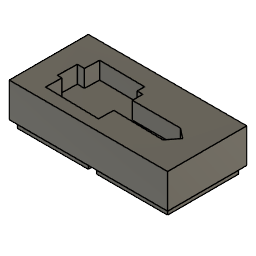
gridfinity module hotend (Autodesk Fusion 360 design; units mm, degrees)
Autodesk Fusion 360 part; units mm, degrees
sketch "Sketch1" plane through (0, 0, 0) normal (0, 0, 1) x (1, 0, 0)
  line L0 (20.75, 20.75) -> (-20.75, 20.75)
  line L1 (-20.75, 20.75) -> (-20.75, -20.75)
  line L2 (-20.75, -20.75) -> (20.75, -20.75)
  line L3 (20.75, -20.75) -> (20.75, 20.75)
  line L4 (20.75, 20.75) -> (-20.75, -20.75) construction
  line L5 (-20.75, 20.75) -> (20.75, -20.75) construction
  dimension "d1" = 41.5
  dimension "d2" = 41.5
  constraint horizontal L0
  constraint perpendicular L0 L1
  constraint parallel L0 L2
  constraint parallel L1 L3
  constraint coincident L4 origin
  constraint coincident L5 origin
  measures "d1" distance of L1.end L2.end
  measures "d2" distance of L0.end L1.end
extrude "Extrude1" add sketch "Sketch1" along normal blind 7 makes body 1
sketch "Sketch2" plane through (0, 20.75, 0) normal (0, 1, 0) x (-1, 0, 0)
  line L0 (-20.75, 0) -> (20.75, 0)
  line L1 (20.75, 0) -> (20.75, 7)
  line L2 (20.75, 7) -> (-20.75, 7)
  line L3 (-20.75, 7) -> (-20.75, 0)
  line L4 (18.6, 0.8) -> (18.6, 2.6)
  line L5 (18.6, 2.6) -> (20.75, 4.75)
  line L6 (17.8, 0) -> (18.6, 0.8)
  line L7 (-18.6, 0.9534) -> (-18.6, 2.7534)
  line L8 (-18.6, 2.7534) -> (-20.75, 4.9034)
  line L9 (-17.8, 0) -> (-18.6, 0.9534)
  line L10 (-20.75, 4.9034) -> (-20.75, 0)
  line L11 (-20.75, 0) -> (-17.8, 0)
  line L12 (20.75, 4.75) -> (20.75, 0)
  line L13 (17.8, 0) -> (20.75, 0)
  constraint coincident L1 L5.end
  constraint coincident L0 L9.start
  constraint coincident L3 L8.end
  constraint coincident L0.start L3.end
  constraint coincident L0.end L1.start
  constraint perpendicular L12 L13
sketch "Sketch3" plane through (-20.75, 0, 0) normal (-1, 0, 0) x (0, -1, 0)
  line L0 (20.75, 7) -> (-20.75, 7)
  line L1 (-20.75, 0) -> (-17.8, 0)
  line L2 (-17.8, 0) -> (-18.6, 0)
  line L3 (-17.8, 0) -> (-18.6, 0.8)
  line L4 (-17.8, 0) -> (-12.38, 0) construction
  line L5 (-18.6, 0.8) -> (-18.6, 2.6)
  line L6 (-18.6, 2.6) -> (-20.75, 4.75)
  line L7 (17.8, 0) -> (18.6, 0.8)
  line L8 (18.6, 0.8) -> (18.6, 2.6)
  line L9 (18.6, 2.6) -> (20.75, 4.75)
  line L10 (20.75, 4.75) -> (20.75, 0)
  line L11 (20.75, 0) -> (17.8, 0)
  line L12 (-20.75, 4.75) -> (-20.75, 0)
  constraint parallel L1 L2
  constraint horizontal L4
  constraint perpendicular L1 L5
  constraint parallel L8 L10
  constraint perpendicular L10 L11
sketch "Sketch4" plane through (0, -20.75, 0) normal (0, -1, 0) x (1, 0, 0)
  line L0 (-20.75, 0) -> (20.75, 0)
  line L1 (20.75, 0) -> (20.75, 7)
  line L2 (20.75, 7) -> (-20.75, 7)
  line L3 (-20.75, 7) -> (-20.75, 0)
  line L4 (-20.75, 0) -> (-17.8, 0)
  line L5 (-17.8, 0) -> (-18.6, 0)
  line L6 (-17.8, 0) -> (-18.6, 0.8)
  line L7 (-17.8, 0) -> (-12.5744, 0) construction
  line L8 (-18.6, 0.8) -> (-18.6, 2.6)
  line L9 (-18.6, 2.6) -> (-20.75, 4.75)
  line L10 (20.75, 0) -> (17.8, 0)
  line L11 (17.8, 0) -> (18.6, 0)
  line L12 (17.8, 0) -> (18.6, 0.8)
  line L13 (18.6, 0.8) -> (18.6, 2.6)
  line L14 (18.6, 2.6) -> (20.75, 4.75)
  constraint coincident L0.start L3.end
  constraint perpendicular L3 L4
  constraint parallel L0 L5
  constraint horizontal L7
  constraint perpendicular L5 L8
  constraint coincident L3 L9.end
  constraint coincident L0.end L1.start
  constraint perpendicular L1 L10
  constraint parallel L10 L11
  constraint perpendicular L10 L13
  constraint coincident L1 L14.end
sketch "Sketch5" plane through (20.75, 0, 0) normal (1, 0, 0) x (0, 1, 0)
  line L0 (-20.75, 0) -> (20.75, 0)
  line L1 (20.75, 0) -> (20.75, 7)
  line L2 (20.75, 7) -> (-20.75, 7)
  line L3 (-20.75, 7) -> (-20.75, 0)
  line L4 (-20.75, 0) -> (-17.8, 0)
  line L5 (-17.8, 0) -> (-18.6, 0)
  line L6 (-17.8, 0) -> (-18.6, 0.8)
  line L7 (-18.6, 0.8) -> (-18.6, 2.6)
  line L8 (-18.6, 2.6) -> (-20.75, 4.75)
  line L9 (20.75, 0) -> (17.8, 0)
  line L10 (17.8, 0) -> (18.6, 0)
  line L11 (18.6, 0.8) -> (18.6, 2.6)
  line L12 (18.6, 2.6) -> (20.75, 4.75)
  line L13 (17.8, 0) -> (18.6, 0.8)
  constraint coincident L0.start L3.end
  constraint perpendicular L3 L4
  constraint parallel L4 L5
  constraint perpendicular L4 L7
  constraint coincident L3 L8.end
  constraint coincident L0.end L1.start
  constraint perpendicular L1 L9
  constraint perpendicular L1 L10
  constraint perpendicular L10 L11
  constraint coincident L1 L12.end
extrude "Extrude2" cut sketch "Sketch5" along normal mid plane 100 contours L0 L3 L4 L5 L6 L7 L8 | L0 L1 L9 L10 L11 L12 L13 bodies 1
extrude "Extrude3" cut sketch "Sketch4" along normal mid plane 100 contours L0 L3 L4 L5 L6 L8 L9 | L0 L1 L10 L11 L12 L13 L14 bodies 1
copy_body "CopyPasteBodies1" bodies 1 makes body 2
move_body "Move1" bodies 2 to x (1, 0, 0) y (0, 1, 0) z (0, 0, 1) at (41.5, 0, 0)
combine "Combine1" operation add target body 1 tool bodies 2
sketch "Sketch6" plane through (0, 0, 7) normal (0, 0, 1) x (-1, 0, 0)
  line L0 (-62.25, -20.75) -> (20.75, -20.75)
  line L1 (20.75, -20.75) -> (20.75, 20.75)
  line L2 (20.75, 20.75) -> (-62.25, 20.75)
  line L3 (-62.25, 20.75) -> (-62.25, -20.75)
  line L4 (10.0352, -4.2687) -> (6.3028, -4.1922)
  line L5 (6.3028, -4.1922) -> (6.0326, -11.9325)
  line L6 (6.0326, -11.9325) -> (-17.7748, -11.649)
  line L7 (-17.7748, -11.649) -> (-17.7285, -7.7618)
  line L8 (-17.7285, -7.7618) -> (-20.7225, -7.7618)
  line L9 (-20.7225, -7.7618) -> (-20.7225, -2.3106)
  line L10 (-20.7225, -2.3106) -> (-45.8884, -2.3106)
  line L11 (-45.8884, -2.3106) -> (-51.1886, 1.836)
  line L12 (-51.1886, 1.836) -> (-46.6533, 7.6332)
  line L13 (-46.6533, 7.6332) -> (-20.3871, 7.0947)
  line L14 (-20.3871, 7.0947) -> (-20.2261, 14.9498)
  line L15 (-20.2261, 14.9498) -> (8.0521, 14.37)
  line L16 (8.0521, 14.37) -> (7.8807, 6.0104)
  line L17 (7.8807, 6.0104) -> (10.245, 5.9619)
  line L18 (10.245, 5.9619) -> (10.0352, -4.2687)
sketch "Sketch7" plane through (0, 0, 0) normal (0, 0, 1) x (1, 0, 0)
  line L0 (-20.75, 20.75) -> (62.25, 20.75)
  line L1 (62.25, 20.75) -> (62.25, -20.75)
  line L2 (62.25, -20.75) -> (-20.75, -20.75)
  line L3 (-20.75, -20.75) -> (-20.75, 20.75)
  constraint horizontal L0
  constraint vertical L1
  constraint horizontal L2
  constraint vertical L3
move_body "Move2" bodies 1 to x (1, 0, 0) y (0, 1, 0) z (0, 0, 1) at (0, 0, -6.75)
extrude "Extrude4" add sketch "Sketch7" along normal blind 16 separate body makes body 3
combine "Combine2" operation add target body 3 tool bodies 1
extrude "Extrude5" cut sketch "Sketch6" along normal blind 16 contours L4 L5 L6 L7 L8 L9 L10 L11 L12 L13 L14 L15 L16 L17 L18 bodies 3
